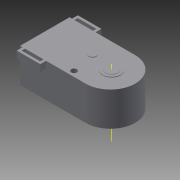
# Autodesk Inventor part: front
Saved by Autodesk Inventor 2014 (Build 180170000, 170)
## iProperties
Created: 2013-06-25
Part Number: front
Material: Generisch
Document SubType Name: Modeling
Designer: Felix
Density: 1 g/cm^3
Appearance: Vorgabe
Author: Felix
Autodesk Inventor part; units mm, degrees
ref_plane "YZ Plane" through (0, 0, 0) normal (1, 0, 0) x (0, 1, 0)
ref_plane "XZ Plane" through (0, 0, 0) normal (0, 1, 0) x (-1, 0, 0)
sketch "Skizze1" plane through (0, 0, 0) normal (0, 0, 1) x (1, 0, 0)
  line L0 (0, 0) -> (36.5, 0)
  line L1 (36.5, 0) -> (36.5, 20)
  line L2 (36.5, 20) -> (0, 20)
  line L3 (0, 20) -> (0, 0)
  dimension "d0" = 36.5
  dimension "d1" = 20
  constraints: 8 end point, 2 parallel, 1 horizontal, 1 perpendicular
  measures "d0" distance of L2.end L1.end
  measures "d1" distance of L1.end L0.end
extrude "Extrusion1" add sketch "Skizze1" along normal blind 13.7
ref_plane "Arbeitsebene1" through (0, 10, 0) normal (0, 1, 0) x (1, 0, 0)
fillet "Rundung1" radius 10 2 edges at (36.5, 20, 6.85) (36.5, 0, 6.85)
sketch "Skizze2" plane through (0, 0, 0) normal (0, 0, -1) x (-1, 0, 0)
  arc A0 (-26.5, 20) -> (-26.5, 0) centre (-26.5, 10) ccw projected
  circle A1 centre (-27, 10) radius 2.5
  circle A2 centre (-27, 10) radius 1.5
  dimension "d5" = 5
  dimension "d6" = 10
  dimension "d7" = 12
  dimension "d8" = 3
  constraints: 2 centre point, 1 coincident
  measures "d5" diameter of A1
  measures "d6" vertical distance of A0.start A1.centre
  measures "d8" diameter of A2
extrude "Extrusion2" add sketch "Skizze2" along normal blind 0.3
sketch "Skizze4" plane through (0, 0, 0) normal (0, 0, -1) x (-1, 0, 0)
  line L0 (0, 0) -> (-26.5, 0) projected
  line L1 (0, 20) -> (0, 0) projected
  circle A0 centre (-19.65, 2.15) radius 1.15
  dimension "d15" = 2.3
  dimension "d16" = 1
  dimension "d17" = 18.5
  constraints: 1 centre point
  measures "d15" diameter of A0
  measures "d16" distance edge to line of A0 L0
  measures "d17" distance edge to line of A0 L1
extrude "Extrusion4" cut sketch "Skizze4" against normal through all
sketch "Skizze5" plane through (0, 0, 0) normal (0, 0, -1) x (-1, 0, 0)
  line L0 (0, 0) -> (-26.5, 0) projected
  line L1 (0, 20) -> (0, 0) projected
  circle A0 centre (-11, 6.5) radius 1.5
  dimension "d21" = 3
  dimension "d23" = 5
  dimension "d24" = 9.5
  constraints: 1 centre point
  measures "d21" diameter of A0
  measures "d23" distance edge to line of A0 L0
  measures "d24" distance edge to line of A0 L1
extrude "Extrusion8" add sketch "Skizze5" along normal blind 0.53
sketch "Skizze6" plane through (0, 0, 0) normal (0, 0, -1) x (-1, 0, 0)
  line L0 (0, 20) -> (0, 0) projected
  line L1 (-26.5, 20) -> (0, 20) projected
  circle A0 centre (-17.6, 11.9) radius 1.5
  dimension "d27" = 3
  dimension "d28" = 6.6
  dimension "d29" = 16.1
  constraints: 1 centre point
  measures "d27" diameter of A0
  measures "d28" distance edge to line of A0 L1
  measures "d29" distance edge to line of A0 L0
extrude "Extrusion5" add sketch "Skizze6" along normal up to surface (0.3 mm away)
sketch "Skizze7" plane through (0, 0, 13.7) normal (0, 0, 1) x (1, 0, 0)
  line L0 (0, 20) -> (0, 0) projected
  line L1 (0, 0) -> (26.5, 0) projected
  circle A0 centre (27, 10) radius 2.5 projected
  circle A1 centre (27, 10) radius 3.65
  circle A2 centre (17.7, 11.6) radius 1.5
  dimension "d34" = 7.3
  dimension "d40" = 3
  dimension "d42" = 10.1
  dimension "d43" = 19.2
  constraints: 2 centre point, 1 coincident
  measures "d34" diameter of A1
  measures "d40" diameter of A2
  measures "d42" distance edge to line of A2 L1
extrude "Extrusion9" add sketch "Skizze7" along normal blind 0.2
sketch "Skizze8" plane through (27, 10, 13.7) normal (0, 0, 1) x (1, 0, 0)
  circle A0 centre (0, 0) radius 2.5 projected
  point P0 (-27, -10)
extrude "Extrusion10" add sketch "Skizze8" along normal blind 0.3
sketch "Skizze11" plane through (0, 20, 13.7) normal (0, 1, 0) x (1, 0, 0)
  line L0 (0, 13.7) -> (0, 0) projected
  line L1 (26.5, 0) -> (0, 0) projected
  line L2 (1, 0) -> (10.5, 0)
  line L3 (10.5, 0) -> (10.5, 2.8)
  line L4 (10.5, 2.8) -> (1, 2.8)
  line L5 (1, 2.8) -> (1, 0)
  dimension "d49" = 9.5
  dimension "d50" = 2.8
  dimension "d51" = 1
  constraints: 8 end point, 2 parallel, 1 horizontal, 1 perpendicular, 1 point on line
  measures "d49" distance of L4.end L3.end
  measures "d50" distance of L3.end L2.end
  measures "d51" distance between parallel lines of L0 L5
extrude "Extrusion11" add sketch "Skizze11" along normal blind 2.35
sketch "Skizze12" plane through (10.5, 20, 10.9) normal (0, 0, -1) x (-1, 0, 0)
  line L0 (9.5, 0) -> (0, 0) projected
  line L1 (9.5, 0) -> (9.5, 2.35) projected
  line L2 (0, 2.35) -> (9.5, 2.35) projected
  line L3 (0, 0) -> (0, 2.35) projected
  line L4 (1, 1.35) -> (8.5, 1.35)
  line L5 (8.5, 1.35) -> (8.5, 0)
  line L6 (8.5, 0) -> (1, 0)
  line L7 (1, 0) -> (1, 1.35)
  point P0 (10.5, -20)
  dimension "d54" = 1
  dimension "d55" = 1
  dimension "d56" = 1
  constraints: 8 end point, 2 parallel, 1 horizontal, 1 perpendicular, 1 point on line
  measures "d54" distance between parallel lines of L2 L4
  measures "d55" distance between parallel lines of L1 L5
  measures "d56" distance between parallel lines of L3 L7
extrude "Extrusion12" cut sketch "Skizze12" against normal through all contours L0 L7 L4 L5
mirror "Spiegeln1" about plane through (0, 10, 0) normal (0, 1, 0) of "Extrusion12", "Extrusion11"
